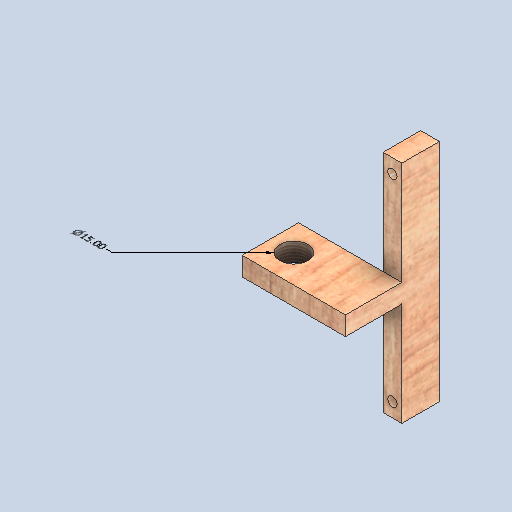
# Autodesk Inventor part: steering_connector[1]
Saved by Autodesk Inventor 2025.2 (Build 292293000, 293)
## iProperties
Created: 2025-02-06
Part Number: steering_connector[1]
Material: Wood (Birch)
Document SubType Name: Modeling
Designer: mpava
Density: 0.55 g/cm^3
Appearance: Birch - Natural Polished
Author: mpava
Autodesk Inventor part; units mm, degrees
ref_plane "YZ Plane" through (0, 0, 0) normal (1, 0, 0) x (0, 1, 0)
ref_plane "XZ Plane" through (0, 0, 0) normal (0, 1, 0) x (-1, 0, 0)
ref_plane "XY Plane" through (0, 0, 0) normal (0, 0, 1) x (1, 0, 0)
sketch "Sketch1" plane through (0, 0, 0) normal (0, 0, 1) x (1, 0, 0)
  line L0 (0, 60) -> (0, -60)
  line L1 (0, -60) -> (-10, -60)
  line L2 (-10, -60) -> (-10, 60)
  line L3 (-10, 60) -> (0, 60)
  point P0 (0, 0)
  dimension "d27" = 120
  dimension "d28" = 10
  constraints: 8 end point, 2 perpendicular, 1 horizontal, 1 vertical
  measures "d27" distance of L0.start L0.end
  measures "d28" distance of L0.end L1.end
extrude "Extrusion1" add sketch "Sketch1" along normal blind 20
sketch "Sketch2" plane through (0, 0, 20) normal (0, 0, 1) x (1, 0, 0)
  line L0 (0, 5) -> (0, -5)
  line L1 (0, -50) -> (0, 50) projected
  line L2 (0, 5) -> (-55, 5)
  line L3 (-55, 5) -> (-55, -5)
  line L4 (-55, -5) -> (0, -5)
  point P0 (0, 0)
  dimension "d5" = 10
  dimension "d6" = 55
  dimension "d7" = 10
  constraints: 8 end point, 1 horizontal, 1 midpoint, 1 perpendicular, 1 point on line
  measures "d5" distance of L0.start L0.end
  measures "d6" distance of L0.start L2.end
  measures "d7" distance of L2.end L3.end
extrude "Extrusion2" add sketch "Sketch2" along normal blind 30
sketch "Sketch3" plane through (-55, 5, 20) normal (0, 1, 0) x (1, 0, 0)
  line L0 (0, 0) -> (0, -30) projected
  line L1 (0, 0) -> (45, 0) projected
  line L2 (0, -30) -> (55, -30) projected
  circle A0 centre (12.5, -15) radius 7.5
  point P0 (55, 20)
  dimension "d12" = 15
  constraints: 1 centre point
  measures "d12" diameter of A0
extrude "Extrusion3" cut sketch "Sketch3" against normal blind 10
sketch "Sketch6" plane through (0, 0, 20) normal (0, 0, 1) x (1, 0, 0)
  circle A0 centre (-5, -52.5) radius 2.5
  circle A1 centre (-5, 52.5) radius 2.5
  point P0 (0, 0)
  dimension "d29" = 5
  dimension "d30" = 5
  constraints: 2 centre point
  measures "d29" diameter of A0
  measures "d30" diameter of A1
extrude "Extrusion6" cut sketch "Sketch6" against normal up to surface (20 mm away)
thread "Thread2" size "M15x1.5" class "6H" standard "ANSI Metric M Profile" length 10
body "Solid1"
